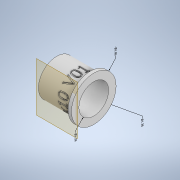
# Autodesk Inventor part: frontPipeDrain-V01
Saved by Autodesk Inventor 2021.1 (Build 251245010, 245A)
## iProperties
Created: 2020-10-20
Part Number: frontPipeDrain-V01
Material: Generic
Document SubType Name: Modeling
Designer: robst
Density: 1 g/cm^3
Appearance: Default
Author: robst
Autodesk Inventor part; units mm, degrees
ref_plane "YZ Plane" through (0, 0, 0) normal (1, 0, 0) x (0, 1, 0)
ref_plane "XZ Plane" through (0, 0, 0) normal (0, 1, 0) x (-1, 0, 0)
sketch "Sketch2" plane through (0, 0, 0) normal (0, 0, 1) x (1, 0, 0)
  line L0 (0, 0) -> (0, 20.955)
  line L1 (0, 20.955) -> (-3.175, 20.955)
  line L2 (-3.175, 20.955) -> (-3.175, 17.145)
  line L3 (-3.175, 17.145) -> (-28.575, 17.145)
  line L4 (-28.575, 17.145) -> (-28.575, 13.97)
  line L5 (-28.575, 13.97) -> (0, 13.97)
  line L6 (-41.91, 0) -> (6.985, 0) projected
  line L7 (-28.575, 13.97) -> (-34.925, 13.97)
  line L8 (-34.925, 13.97) -> (-34.925, 17.145)
  line L9 (-34.925, 17.145) -> (-28.575, 17.145)
  line L10 (-28.575, 17.145) -> (-28.575, 13.97)
  dimension "d0" = 20.955
  dimension "d1" = 13.97
  dimension "d2" = 3.175
  dimension "d3" = 25.4
  dimension "d5" = 17.145
  dimension "d6" = 6.35
  constraints: 20 end point, 6 perpendicular, 2 parallel, 1 collinear, 1 horizontal, 1 point on line, 1 vertical
  measures "d0" distance from line of L0.start L1
  measures "d1" distance from line of L5 L0.start
  measures "d2" distance between parallel lines of L0 L2
  measures "d3" distance from line of L3.end L2
  measures "d5" distance from line of L3 L0.start
  measures "d6" distance between parallel lines of L8 L4
revolve "Revolution1" add sketch "Sketch2" angle 360 about axis through (-10, 0, 0) along (1, 0, 0)
ref_plane "Work Plane1" through (-19.05, 0, 17.145) normal (0, 0, 1) x (1, 0, 0)
sketch "Sketch5" plane through (-19.05, 0, 17.145) normal (0, 0, 1) x (1, 0, 0)
  line L0 (-15.875, 17.145) -> (15.875, 17.145) projected
  line L1 (-15.875, -17.145) -> (15.875, -17.145) projected
  line L2 (15.875, -20.955) -> (15.875, 20.955) projected
  line L3 (6.985, -17.145) -> (6.985, 17.145) construction
  spline S0 degree 2 poles (4.6292, -27.0266) (5.2128, -27.0266) (6.1277, -27.4156) (6.4735, -27.7398) knots 0 0 0 1 2 2 2
  spline S1 degree 2 poles (6.4735, -27.7398) (6.8193, -28.0568) (7.4028, -28.8781) (7.6766, -29.332) knots 0 0 0 1 2 2 2
  line L4 (7.6766, -29.332) -> (9.0382, -29.332)
  line L5 (9.0382, -29.332) -> (9.0382, -30.3982)
  line L6 (9.0382, -30.3982) -> (7.2155, -30.3982)
  spline S2 degree 2 poles (7.2155, -30.3982) (7.0138, -30.0668) (6.4519, -29.1735) (6.2069, -28.9213) knots 0 0 0 1 2 2 2
  spline S3 degree 2 poles (6.2069, -28.9213) (5.8972, -28.6043) (5.1767, -28.2441) (4.7157, -28.2441) knots 0 0 0 1 2 2 2
  spline S4 degree 2 poles (4.7157, -28.2441) (4.0457, -28.2441) (3.3829, -29.0942) (3.3829, -29.7714) knots 0 0 0 1 2 2 2
  spline S5 degree 2 poles (3.3829, -29.7714) (3.3829, -30.3694) (3.7791, -31.4212) (3.9953, -31.7526) knots 0 0 0 1 2 2 2
  line L7 (3.9953, -31.7526) -> (3.9953, -31.8174)
  line L8 (3.9953, -31.8174) -> (2.7777, -31.8174)
  spline S6 degree 2 poles (2.7777, -31.8174) (2.6192, -31.4212) (2.3599, -30.2037) (2.3599, -29.6561) knots 0 0 0 1 2 2 2
  spline S7 degree 2 poles (2.3599, -29.6561) (2.3599, -28.4314) (3.6062, -27.0266) (4.6292, -27.0266) knots 0 0 0 1 2 2 2
  line L9 (11.43, -29.2383) -> (11.43, -30.4486)
  line L10 (11.43, -30.4486) -> (10.1693, -30.4486)
  line L11 (10.1693, -30.4486) -> (10.1693, -29.2383)
  line L12 (10.1693, -29.2383) -> (11.43, -29.2383)
  line L13 (11.43, -24.1161) -> (11.43, -25.5425)
  line L14 (11.43, -25.5425) -> (9.7298, -25.5425)
  line L15 (9.7298, -25.5425) -> (9.7298, -24.1161)
  line L16 (9.7298, -24.1161) -> (11.43, -24.1161)
  spline S8 degree 2 poles (4.6292, -17.5315) (5.2128, -17.5315) (6.1277, -17.9205) (6.4735, -18.2447) knots 0 0 0 1 2 2 2
  spline S9 degree 2 poles (6.4735, -18.2447) (6.8193, -18.5617) (7.4028, -19.3829) (7.6766, -19.8368) knots 0 0 0 1 2 2 2
  line L17 (7.6766, -19.8368) -> (9.0382, -19.8368)
  line L18 (9.0382, -19.8368) -> (9.0382, -20.903)
  line L19 (9.0382, -20.903) -> (7.2155, -20.903)
  spline S10 degree 2 poles (7.2155, -20.903) (7.0138, -20.5716) (6.4519, -19.6783) (6.2069, -19.4262) knots 0 0 0 1 2 2 2
  spline S11 degree 2 poles (6.2069, -19.4262) (5.8972, -19.1092) (5.1767, -18.749) (4.7157, -18.749) knots 0 0 0 1 2 2 2
  spline S12 degree 2 poles (4.7157, -18.749) (4.0457, -18.749) (3.3829, -19.5991) (3.3829, -20.2763) knots 0 0 0 1 2 2 2
  spline S13 degree 2 poles (3.3829, -20.2763) (3.3829, -20.8742) (3.7791, -21.926) (3.9953, -22.2574) knots 0 0 0 1 2 2 2
  line L20 (3.9953, -22.2574) -> (3.9953, -22.3223)
  line L21 (3.9953, -22.3223) -> (2.7777, -22.3223)
  spline S14 degree 2 poles (2.7777, -22.3223) (2.6192, -21.926) (2.3599, -20.7085) (2.3599, -20.161) knots 0 0 0 1 2 2 2
  spline S15 degree 2 poles (2.3599, -20.161) (2.3599, -18.9363) (3.6062, -17.5315) (4.6292, -17.5315) knots 0 0 0 1 2 2 2
  line L22 (11.43, -19.7431) -> (11.43, -20.9535)
  line L23 (11.43, -20.9535) -> (10.1693, -20.9535)
  line L24 (10.1693, -20.9535) -> (10.1693, -19.7431)
  line L25 (10.1693, -19.7431) -> (11.43, -19.7431)
  spline S16 degree 2 poles (4.6292, -11.7393) (5.2128, -11.7393) (6.1277, -12.1283) (6.4735, -12.4525) knots 0 0 0 1 2 2 2
  spline S17 degree 2 poles (6.4735, -12.4525) (6.8193, -12.7695) (7.4028, -13.5907) (7.6766, -14.0446) knots 0 0 0 1 2 2 2
  line L26 (7.6766, -14.0446) -> (9.0382, -14.0446)
  line L27 (9.0382, -14.0446) -> (9.0382, -15.1108)
  line L28 (9.0382, -15.1108) -> (7.2155, -15.1108)
  spline S18 degree 2 poles (7.2155, -15.1108) (7.0138, -14.7794) (6.4519, -13.8861) (6.2069, -13.634) knots 0 0 0 1 2 2 2
  spline S19 degree 2 poles (6.2069, -13.634) (5.8972, -13.317) (5.1767, -12.9568) (4.7157, -12.9568) knots 0 0 0 1 2 2 2
  spline S20 degree 2 poles (4.7157, -12.9568) (4.0457, -12.9568) (3.3829, -13.8069) (3.3829, -14.4841) knots 0 0 0 1 2 2 2
  spline S21 degree 2 poles (3.3829, -14.4841) (3.3829, -15.082) (3.7791, -16.1338) (3.9953, -16.4652) knots 0 0 0 1 2 2 2
  line L29 (3.9953, -16.4652) -> (3.9953, -16.5301)
  line L30 (3.9953, -16.5301) -> (2.7777, -16.5301)
  spline S22 degree 2 poles (2.7777, -16.5301) (2.6192, -16.1338) (2.3599, -14.9163) (2.3599, -14.3688) knots 0 0 0 1 2 2 2
  spline S23 degree 2 poles (2.3599, -14.3688) (2.3599, -13.1441) (3.6062, -11.7393) (4.6292, -11.7393) knots 0 0 0 1 2 2 2
  line L31 (11.43, -13.951) -> (11.43, -15.1613)
  line L32 (11.43, -15.1613) -> (10.1693, -15.1613)
  line L33 (10.1693, -15.1613) -> (10.1693, -13.951)
  line L34 (10.1693, -13.951) -> (11.43, -13.951)
  line L35 (11.43, -5.3924) -> (11.43, -6.7684)
  line L36 (11.43, -6.7684) -> (8.9229, -8.3893)
  line L37 (8.9229, -8.3893) -> (11.43, -10.0535)
  line L38 (11.43, -10.0535) -> (11.43, -11.3286)
  line L39 (11.43, -11.3286) -> (8.1233, -9.0161)
  line L40 (8.1233, -9.0161) -> (4.7589, -11.307)
  line L41 (4.7589, -11.307) -> (4.7589, -9.931)
  line L42 (4.7589, -9.931) -> (7.2444, -8.3173)
  line L43 (7.2444, -8.3173) -> (4.7589, -6.6675)
  line L44 (4.7589, -6.6675) -> (4.7589, -5.3924)
  line L45 (4.7589, -5.3924) -> (8.0512, -7.6905)
  line L46 (8.0512, -7.6905) -> (11.43, -5.3924)
  line L47 (11.43, 0.3494) -> (11.43, -3.9875)
  line L48 (11.43, -3.9875) -> (10.5223, -3.9875)
  line L49 (10.5223, -3.9875) -> (10.5223, -2.3738)
  line L50 (10.5223, -2.3738) -> (4.5644, -2.3738)
  line L51 (4.5644, -2.3738) -> (4.5644, -3.9875)
  line L52 (4.5644, -3.9875) -> (3.7503, -3.9875)
  spline S24 degree 2 poles (3.7503, -3.9875) (3.7503, -3.0726) (3.2316, -2.2081) (2.5112, -2.1505) knots 0 0 0 1 2 2 2
  line L53 (2.5112, -2.1505) -> (2.5112, -1.2283)
  line L54 (2.5112, -1.2283) -> (10.5223, -1.2283)
  line L55 (10.5223, -1.2283) -> (10.5223, 0.3494)
  line L56 (10.5223, 0.3494) -> (11.43, 0.3494)
  spline S25 degree 2 poles (6.985, 7.5176) (9.3768, 7.5176) (11.6173, 6.1272) (11.6173, 4.6791) knots 0 0 0 1 2 2 2
  spline S26 degree 2 poles (11.6173, 4.6791) (11.6173, 3.2095) (9.3336, 1.8335) (6.9922, 1.8335) knots 0 0 0 1 2 2 2
  spline S27 degree 2 poles (6.9922, 1.8335) (4.586, 1.8335) (2.3599, 3.2239) (2.3599, 4.6791) knots 0 0 0 1 2 2 2
  spline S28 degree 2 poles (2.3599, 4.6791) (2.3599, 6.1416) (4.6652, 7.5176) (6.985, 7.5176) knots 0 0 0 1 2 2 2
  spline S29 degree 2 poles (9.6938, 5.9903) (9.2543, 6.1632) (7.8999, 6.3073) (6.985, 6.3073) knots 0 0 0 1 2 2 2
  spline S30 degree 2 poles (6.985, 6.3073) (6.0701, 6.3073) (4.7229, 6.1632) (4.269, 5.9831) knots 0 0 0 1 2 2 2
  spline S31 degree 2 poles (4.269, 5.9831) (3.8151, 5.803) (3.3469, 5.1762) (3.3469, 4.6791) knots 0 0 0 1 2 2 2
  spline S32 degree 2 poles (3.3469, 4.6791) (3.3469, 4.182) (3.8151, 3.5409) (4.2834, 3.3536) knots 0 0 0 1 2 2 2
  spline S33 degree 2 poles (4.2834, 3.3536) (4.7373, 3.1735) (6.1205, 3.0438) (6.9922, 3.0438) knots 0 0 0 1 2 2 2
  spline S34 degree 2 poles (6.9922, 3.0438) (7.9288, 3.0438) (9.1823, 3.159) (9.6722, 3.3464) knots 0 0 0 1 2 2 2
  spline S35 degree 2 poles (9.6722, 3.3464) (10.1332, 3.5193) (10.6303, 4.1604) (10.6303, 4.6791) knots 0 0 0 1 2 2 2
  spline S36 degree 2 poles (10.6303, 4.6791) (10.6303, 5.169) (10.1621, 5.8102) (9.6938, 5.9903) knots 0 0 0 1 2 2 2
  line L57 (2.54, 19.174) -> (11.43, 16.1122)
  line L58 (11.43, 16.1122) -> (11.43, 14.8371)
  line L59 (11.43, 14.8371) -> (2.54, 11.7753)
  line L60 (2.54, 11.7753) -> (2.54, 13.0432)
  line L61 (2.54, 13.0432) -> (9.9243, 15.5071)
  line L62 (9.9243, 15.5071) -> (2.54, 17.9709)
  line L63 (2.54, 17.9709) -> (2.54, 19.174)
  spline S37 degree 2 poles (6.985, 25.4057) (9.3768, 25.4057) (11.6173, 24.0152) (11.6173, 22.5672) knots 0 0 0 1 2 2 2
  spline S38 degree 2 poles (11.6173, 22.5672) (11.6173, 21.0975) (9.3336, 19.7215) (6.9922, 19.7215) knots 0 0 0 1 2 2 2
  spline S39 degree 2 poles (6.9922, 19.7215) (4.586, 19.7215) (2.3599, 21.1119) (2.3599, 22.5672) knots 0 0 0 1 2 2 2
  spline S40 degree 2 poles (2.3599, 22.5672) (2.3599, 24.0297) (4.6652, 25.4057) (6.985, 25.4057) knots 0 0 0 1 2 2 2
  spline S41 degree 2 poles (9.6938, 23.8784) (9.2543, 24.0513) (7.8999, 24.1954) (6.985, 24.1954) knots 0 0 0 1 2 2 2
  spline S42 degree 2 poles (6.985, 24.1954) (6.0701, 24.1954) (4.7229, 24.0513) (4.269, 23.8712) knots 0 0 0 1 2 2 2
  spline S43 degree 2 poles (4.269, 23.8712) (3.8151, 23.6911) (3.3469, 23.0643) (3.3469, 22.5672) knots 0 0 0 1 2 2 2
  spline S44 degree 2 poles (3.3469, 22.5672) (3.3469, 22.0701) (3.8151, 21.4289) (4.2834, 21.2416) knots 0 0 0 1 2 2 2
  spline S45 degree 2 poles (4.2834, 21.2416) (4.7373, 21.0615) (6.1205, 20.9318) (6.9922, 20.9318) knots 0 0 0 1 2 2 2
  spline S46 degree 2 poles (6.9922, 20.9318) (7.9288, 20.9318) (9.1823, 21.0471) (9.6722, 21.2344) knots 0 0 0 1 2 2 2
  spline S47 degree 2 poles (9.6722, 21.2344) (10.1332, 21.4073) (10.6303, 22.0485) (10.6303, 22.5672) knots 0 0 0 1 2 2 2
  spline S48 degree 2 poles (10.6303, 22.5672) (10.6303, 23.0571) (10.1621, 23.6983) (9.6938, 23.8784) knots 0 0 0 1 2 2 2
  line L64 (11.43, 31.5797) -> (11.43, 27.2427)
  line L65 (11.43, 27.2427) -> (10.5223, 27.2427)
  line L66 (10.5223, 27.2427) -> (10.5223, 28.8565)
  line L67 (10.5223, 28.8565) -> (4.5644, 28.8565)
  line L68 (4.5644, 28.8565) -> (4.5644, 27.2427)
  line L69 (4.5644, 27.2427) -> (3.7503, 27.2427)
  spline S49 degree 2 poles (3.7503, 27.2427) (3.7503, 28.1577) (3.2316, 29.0222) (2.5112, 29.0798) knots 0 0 0 1 2 2 2
  line L70 (2.5112, 29.0798) -> (2.5112, 30.0019)
  line L71 (2.5112, 30.0019) -> (10.5223, 30.0019)
  line L72 (10.5223, 30.0019) -> (10.5223, 31.5797)
  line L73 (10.5223, 31.5797) -> (11.43, 31.5797)
  point P0 (19.05, 0)
  dimension "d35" = 8.89
  constraints: 2 end point, 2 point on line, 1 perpendicular, 1 vertical
  measures "d35" distance between parallel lines of L3 L2
emboss "Emboss1" sketch "Sketch5" operation cut depth 1.27 direction (0, 0, -1) wrap yes faces at (-13.7583, 16.923, -2.7503)
sketch "Sketch4" plane through (0, 0, 0) normal (0, 0, 1) x (1, 0, 0)
  line L0 (-38.4127, 15.1606) -> (-37.6784, 13.8887)
  line L1 (-37.2516, 13.8887) -> (-36.5173, 15.1606)
  arc A0 (-37.6784, 13.8887) -> (-37.2516, 13.8887) centre (-37.465, 14.0119) ccw
  line L2 (-39.0573, 15.1606) -> (-40.3283, 12.9592)
  line L3 (-35.8727, 15.1606) -> (-33.7873, 11.5486)
  arc A1 (-38.4127, 15.1606) -> (-39.0573, 15.1606) centre (-38.735, 14.9745) ccw
  arc A2 (-35.8727, 15.1606) -> (-36.5173, 15.1606) centre (-36.195, 14.9745) ccw
  line L4 (-38.735, 15.3467) -> (-36.195, 15.3467)
  line L5 (-34.925, -17.145) -> (-34.925, 17.145) construction
  line L6 (-34.925, 0) -> (-40.005, 0) construction
  line L7 (-40.3283, 12.9592) -> (-40.3283, 16.2117) construction
  point P0 (0, 0)
  dimension "d10" = 60
  dimension "d11" = 0.2464
  dimension "d12" = 60
  dimension "d13" = 60
  dimension "d15" = 2.54
  dimension "d16" = 5.08
  dimension "d17" = 1.27
  dimension "d18" = 15.3467
  dimension "d19" = 13.7655
  dimension "d20" = 30
  constraints: 14 end point, 8 point on circle, 6 tangent, 3 centre point, 2 horizontal, 1 equal radius, 1 midpoint, 1 vertical
  measures "d10" angle of L1 L0
  measures "d11" radius of A0
  measures "d12" angle of L0 L2
  measures "d13" angle of L3 L1
  measures "d15" distance of A2.centre A1.centre
  measures "d16" distance from line of L6.end L5
  measures "d17" distance from line of A2.centre L5
  measures "d18" distance between parallel lines of L4 L6
  measures "d19" distance edge to line of A0 L6
  measures "d20" angle of L7 L2
equation "\"d0\" = flangeRadius"
equation "\"d1\" = pipeRadius"
equation "\"d2\" = flangeThickness"
equation "\"d3\" = houseWallThickness"
equation "\"d5\" = houseHoleRadius"
equation "\"d6\" = allowanceForThreadRing"
equation "\"d10\" = threadAngle"
equation "\"d11\" = a1RootRadius"
equation "\"d12\" = threadAngle"
equation "\"d13\" = threadAngle"
equation "\"d15\" = pitch"
equation "\"d16\" = 2 * pitch"
equation "\"d17\" = 0.5 * pitch"
equation "\"d18\" = 0.5 * a1MajorDiameter"
equation "\"d19\" = 0.5 * a1MinorDiameter"
equation "\"d20\" = 0.5 * threadAngle"
equation "\"houseHoleDiameter\" = 34.29"
equation "\"pipeDiameter\" = 27.94"
equation "\"houseHoleRadius\" = 0.5 * houseHoleDiameter"
equation "\"pipeRadius\" = 0.5 * pipeDiameter"
equation "\"houseWallThickness\" = 25.4"
equation "\"allowanceForThreadRing\" = 6.35"
equation "\"threadDepth\" = 15.875"
equation "\"flangeDiameter\" = 41.91"
equation "\"flangeRadius\" = 0.5 * flangeDiameter"
equation "\"a1MajorDiameter\" = 30.69336"
equation "\"a1MinorDiameter\" = 27.53106"
equation "\"a1RootRadius\" = 0.24638"
equation "\"threadAngle\" = 60deg"
equation "\"flangeThickness\" = 3.175"
equation "\"pitch\" = 2.54"
body "Solid1"
